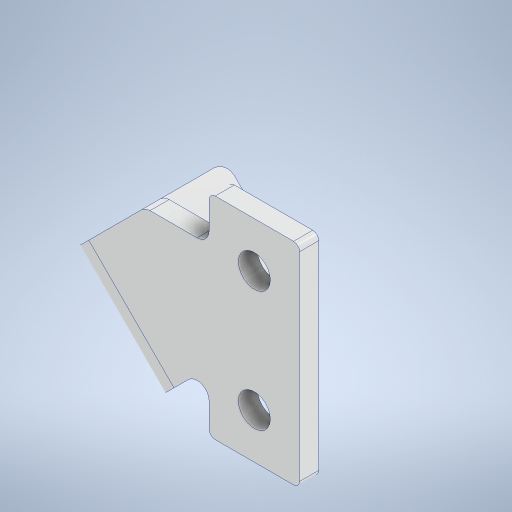
# Autodesk Inventor part: External Frame Corner Bracket
Saved by Autodesk Inventor 2024 (Build 280153000, 153)
## iProperties
Created: 2024-12-02
Part Number: External Frame Corner Bracket
Material: Aluminum 6061
Document SubType Name: Sheet Metal
Designer: Ishaan
Density: 2.7 g/cm^3
Sheet Metal Rule: SendCutSend_1-8_Alu
Appearance: Aluminum - Flat
Author: Ishaan
Autodesk Inventor part; units mm, degrees
ref_plane "YZ Plane" through (0, 0, 0) normal (1, 0, 0) x (0, 1, 0)
ref_plane "XZ Plane" through (0, 0, 0) normal (0, 1, 0) x (-1, 0, 0)
ref_plane "XY Plane" through (0, 0, 0) normal (0, 0, 1) x (1, 0, 0)
sketch "Sketch1" plane through (0, 0, 0) normal (0, 0, 1) x (1, 0, 0)
  line L0 (0, -21.2132) -> (-21.2132, 0) construction
  line L1 (-21.2132, 0) -> (0, 21.2132) construction
  line L2 (0, 21.2132) -> (21.2132, 0) construction
  line L3 (21.2132, 0) -> (0, -21.2132) construction
  line L4 (0, -21.2132) -> (0, 21.2132) construction
  line L5 (-21.2132, 0) -> (21.2132, 0) construction
  line L6 (43, 4) -> (28, 4)
  line L7 (28, 4) -> (28, 39)
  line L8 (28, 39) -> (43, 39)
  line L9 (43, 39) -> (43, 4)
  line L10 (43, 4) -> (28, 39) construction
  line L11 (28, 4) -> (43, 39) construction
  line L12 (35.5, 11.5) -> (35.5, 31.5) construction
  line L13 (17.6777, 3.5355) -> (3.5355, 17.6777)
  line L14 (3.5355, 17.6777) -> (17.3579, 31.5)
  line L15 (17.3579, 31.5) -> (28, 31.5)
  line L16 (17.6777, 3.5355) -> (25.6421, 11.5)
  line L17 (25.6421, 11.5) -> (28, 11.5)
  line L18 (28, 11.5) -> (28, 31.5)
  point P0 (0, 0)
  point P1 (35.5, 21.5)
  point P2 (0, 0)
  point P3 (0, 0)
  point P4 (35.5, 21.5)
  point P5 (43, 21.5)
  point P6 (10.6066, 10.6066)
  point P7 (28, 21.5)
  dimension "d0" = 30
  dimension "d1" = 28
  dimension "d2" = 21.5
  dimension "d3" = 35
  dimension "d5" = 20
  dimension "d6" = 7.5
  dimension "d7" = 7.5
  dimension "d8" = 7.5
  dimension "d11" = 20
  dimension "d12" = 20
  constraints: 38 end point, 12 midpoint, 5 parallel, 5 perpendicular, 4 point on line, 2 horizontal, 2 vertical, 1 collinear, 1 horizontal alignment
  measures "d0" distance of L0.end L1.end
  measures "d1" distance from line of L7 point (0, 0)
  measures "d2" vertical distance of point (35.5, 21.5) point (0, 0)
  measures "d3" distance of L8.end L6.start
  measures "d5" distance of L12.start L12.end
  measures "d6" distance between parallel lines of L9 L12
  measures "d7" distance from line of L8 L12.end
  measures "d8" distance between parallel lines of L12 L7
  measures "d11" distance between parallel lines of L14 L16
  measures "d12" distance between parallel lines of L15 L17
extrude "Plate2" add sketch "Sketch1" against normal blind 3.175
sketch "Sketch2" plane through (5.7806, 19.9227, 0) normal (-0.7071068, -0.7071068, 0) x (0.7071068, -0.7071068, 0)
  line L0 (20, 0) -> (0, 0)
  line L1 (0, 0) -> (0, -25)
  line L2 (0, -25) -> (20, -25)
  line L3 (20, -25) -> (20, 0)
  constraints: 6 end point, 1 horizontal, 1 perpendicular, 1 vertical
edge flange "Flange1" height 25 angle 90 thickness 3.175 bend radius 3.175 thickness toward (-0.7071068, -0.7071068, 0) relief tear relief width 3.175 relief depth 1.5875 edges at (10.6066, 10.6066, -3.175) wall of the first edge with corners at (19.9227, 5.7806, 0) (5.7806, 19.9227, 0) (5.7806, 19.9227, -25) (19.9227, 5.7806, -25)
bend "Bend1"
corner "Corner1"
fillet "Fillet1" radius 2 4 edges at (25.6421, 11.5, -1.5875) (28, 11.5, -1.5875) (28, 31.5, -1.5875) (17.3579, 31.5, -1.5875)
sketch "Sketch3" plane through (3.5355, 17.6777, -6.35) normal (-0.7071068, -0.7071068, 0) x (-0.7071068, 0.7071068, 0)
  line L0 (0, -1.35) -> (-20, -1.35) construction
  line L1 (-20, -1.35) -> (-20, 18.65) construction
  line L2 (-20, 18.65) -> (0, 18.65) construction
  line L3 (0, 18.65) -> (0, -1.35) construction
  line L4 (0, -1.35) -> (-20, 18.65) construction
  line L5 (-20, -1.35) -> (0, 18.65) construction
  point P0 (-10, -6.35)
  point P1 (-10, 8.65)
  constraints: 12 end point, 2 coincident, 2 midpoint, 2 parallel, 2 perpendicular, 1 horizontal
hole "Hole2" at (10.6066, 10.6066, -15) direction (0.7071068, 0.7071068, 0) diameter 6.3 end through all
fillet "Fillet2" radius 2 2 edges at (4.6581, 18.8002, -25) (18.8002, 4.6581, -25)
fillet "Fillet3" radius 1 4 edges at (28, 4, -1.5875) (28, 39, -1.5875) (43, 4, -1.5875) (43, 39, -1.5875)
hole "Hole1" at (35.5, 31.5, 0) at (35.5, 11.5, 0) direction (0, 0, -1) diameter 5.3 end through all
equation "\"d6\" = d7"
equation "\"d8\" = d6"
equation "\"d12\" = d11"
equation "\"d32\" = Thickness"
equation "\"d13\" = Thickness"
equation "\"d14\" = BendReliefWidth"
equation "\"d15\" = BendReliefDepth"
equation "\"d16\" = MinimumRemnant"
equation "\"d17\" = TransitionRadius"
equation "\"d20\" = BendRadius"
equation "\"d21\" = CornerReliefSize"
equation "\"d22\" = GapSize"
equation "\"d23\" = JacobiRadiusSize"
equation "\"BendReliefWidth\" = Thickness"
equation "\"BendReliefDepth\" = 0.5 * Thickness"
equation "\"CornerReliefSize\" = 4 * Thickness"
equation "\"MinimumRemnant\" = 2 * Thickness"
equation "\"TransitionRadius\" = BendRadius"
equation "\"JacobiRadiusSize\" = BendRadius"
equation "\"GapSize\" = Thickness"
equation "\"Thickness\" = 3.175"
equation "\"BendRadius\" = 3.175"
body "Solid2"
